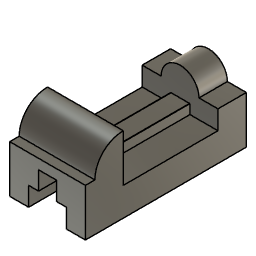
Robocon_Task1C_2 v1 (Autodesk Fusion 360 design; units mm, degrees)
Autodesk Fusion 360 part; units mm, degrees
sketch "Sketch1" plane through (0, 0, 0) normal (0, 0, 1) x (1, 0, 0) in component "Component"
  line L0 (40, -85) -> (-40, -85)
  line L1 (-40, -85) -> (-40, 85)
  line L2 (-40, 85) -> (40, 85)
  line L3 (40, 85) -> (40, -85)
  line L4 (40, -85) -> (-40, 85) construction
  line L5 (-40, -85) -> (40, 85) construction
  dimension "d1" = 80
  dimension "d2" = 170
  constraint horizontal L0
  constraint perpendicular L0 L1
  constraint parallel L0 L2
  constraint parallel L1 L3
  constraint coincident L4 origin
  constraint coincident L5 origin
  measures "d1" distance of L1.end L2.end
  measures "d2" distance of L0.end L1.end
extrude "Extrude1" add sketch "Sketch1" along normal blind 30 in component "Component"
sketch "Sketch2" plane through (0, 0, 30) normal (0, 0, 1) x (-1, 0, 0) in component "Component"
  line L0 (-40, -85) -> (40, -85)
  line L1 (40, -85) -> (40, 85)
  line L2 (40, 85) -> (-40, 85)
  line L3 (-40, 85) -> (-40, -85)
  line L4 (40, 75) -> (-40, 75)
  dimension "d5" = 10
  constraint coincident L1 L4.start
  constraint coincident L3 L4.end
  constraint perpendicular L3 L4
  measures "d5" distance of L2 L4
extrude "Extrude2" add sketch "Sketch2" along normal blind 20 contours L1 L2 L3 L4 in component "Component"
sketch "Sketch3" plane through (0, -85, 0) normal (0, -1, 0) x (1, 0, 0) in component "Component"
  line L0 (-40, 0) -> (40, 0)
  line L1 (40, 0) -> (40, 50)
  line L2 (40, 50) -> (-40, 50)
  line L3 (-40, 50) -> (-40, 0)
  line L4 (-20, 0) -> (-20, 20)
  line L5 (-20, 20) -> (-10, 20)
  line L6 (-10, 20) -> (-10, 40)
  line L7 (-10, 40) -> (10, 40)
  line L8 (10, 40) -> (10, 20)
  line L9 (10, 20) -> (20, 20)
  line L10 (20, 20) -> (20, 0)
  constraint coincident L0 L4.start
  constraint perpendicular L0 L4
  constraint perpendicular L4 L5
  constraint perpendicular L5 L6
  constraint perpendicular L6 L7
  constraint perpendicular L7 L8
  constraint perpendicular L8 L9
  constraint coincident L0 L10.end
  constraint perpendicular L0 L10
sketch "Sketch4" plane through (0, 0, 30) normal (0, 0, 1) x (-1, 0, 0) in component "Component"
  line L0 (40, 75) -> (-40, 75)
  line L1 (-40, 75) -> (-40, -85)
  line L2 (-40, -85) -> (40, -85)
  line L3 (40, -85) -> (40, 75)
  line L4 (40, -55) -> (-40, -55)
  dimension "d10" = 30
  constraint coincident L3 L4.start
  constraint perpendicular L3 L4
  measures "d10" distance of L2 L4
extrude "Extrude4" add sketch "Sketch4" along normal blind 40 contours L1 L2 L3 L4 in component "Component"
sketch "Sketch5" plane through (0, 55, 0) normal (0, -1, 0) x (1, 0, 0) in component "Component"
  line L0 (-40, 30) -> (40, 30)
  line L1 (40, 30) -> (40, 70)
  line L2 (40, 70) -> (-40, 70)
  line L3 (-40, 70) -> (-40, 30)
  circle A0 centre (0, 50) radius 20
  line L4 (-40, 50) -> (40, 50)
  dimension "d13" = 40
  dimension "d14" = 20
  constraint tangent L2 A0
  constraint midpoint L3 L4.start
  constraint midpoint L1 L4.end
  measures "d13" distance of L1 A0.centre
  measures "d14" distance of L2 A0.centre
extrude "Extrude5" cut sketch "Sketch5" against normal up to surface (30 mm away) contours L2 L3 A0 L4 | L1 L2 A0 L4 in component "Component"
sketch "Sketch6" plane through (0, 0, 30) normal (0, 0, 1) x (-1, 0, 0) in component "Component"
  line L0 (-40, -55) -> (40, -55)
  line L1 (40, -55) -> (40, 75)
  line L2 (40, 75) -> (-40, 75)
  line L3 (-40, 75) -> (-40, -55)
  line L4 (-40, 45) -> (40, 45)
  dimension "d17" = 30
  constraint coincident L3 L4.start
  constraint coincident L1 L4.end
  constraint perpendicular L1 L4
  measures "d17" distance of L2 L4
extrude "Extrude6" add sketch "Sketch6" along normal blind 50 contours L1 L2 L3 L4 in component "Component"
sketch "Sketch7" plane through (40, 0, 0) normal (1, 0, 0) x (0, 1, 0) in component "Component"
  line L0 (85, 50) -> (55, 50)
  line L1 (55, 50) -> (55, 30)
  line L2 (55, 30) -> (-45, 30)
  line L3 (-45, 30) -> (-45, 80)
  line L4 (-45, 80) -> (-75, 80)
  line L5 (-75, 80) -> (-75, 50)
  line L6 (-75, 50) -> (-85, 50)
  line L7 (-85, 50) -> (-85, 0)
  line L8 (-85, 0) -> (85, 0)
  line L9 (85, 0) -> (85, 50)
  circle A0 centre (-45, 50) radius 30
  dimension "d20" = 60
  constraint coincident L3 A0.centre
  constraint coincident L5.end A0
  measures "d20" diameter of A0
extrude "Extrude7" cut sketch "Sketch7" against normal up to surface (80 mm away) contours L4 L5 A0 in component "Component"
sketch "Sketch8" plane through (0, -85, 0) normal (0, -1, 0) x (1, 0, 0) in component "Component"
  line L0 (-40, 0) -> (40, 0)
  line L1 (40, 0) -> (40, 50)
  line L2 (40, 50) -> (-40, 50)
  line L3 (-40, 50) -> (-40, 0)
  line L4 (-20, 0) -> (-20, 20)
  line L5 (-20, 20) -> (-10, 20)
  line L6 (10, 20) -> (20, 20)
  line L7 (20, 20) -> (20, 0)
  line L8 (10, 20) -> (-10, 20)
  constraint coincident L0 L4.start
  constraint perpendicular L0 L4
  constraint perpendicular L4 L5
  constraint coincident L0 L7.end
  constraint perpendicular L0 L7
  constraint parallel L5 L8
extrude "Extrude8" cut sketch "Sketch8" against normal up to surface (170 mm away) contours L0 L4 L5 L6 L7 L8 in component "Component"
sketch "Sketch10" plane through (0, 0, 30) normal (0, 0, 1) x (-1, 0, 0) in component "Component"
  line L0 (40, 45) -> (-40, 45)
  line L1 (-40, 45) -> (-40, -55)
  line L2 (-40, -55) -> (40, -55)
  line L3 (40, -55) -> (40, 45)
  line L4 (-10.4269, -55) -> (-10.4269, 45)
  line L5 (9.8376, 45) -> (9.8376, -55)
  constraint coincident L2 L4.start
  constraint coincident L0 L4.end
  constraint perpendicular L0 L4
  constraint coincident L0 L5.start
  constraint coincident L2 L5.end
  constraint perpendicular L2 L5
extrude "Extrude9" add sketch "Sketch10" along normal blind 10 contours L0 L2 L4 L5 in component "Component"
sketch "Sketch13" plane through (0, -85, 0) normal (0, -1, 0) x (1, 0, 0) in component "Component"
  line L0 (-20, 0) -> (-20, 20)
  line L1 (-20, 20) -> (20, 20)
  line L2 (20, 20) -> (20, 0)
  line L3 (20, 0) -> (40, 0)
  line L4 (40, 0) -> (40, 50)
  line L5 (40, 50) -> (-40, 50)
  line L6 (-40, 50) -> (-40, 0)
  line L7 (-40, 0) -> (-20, 0)
  line L8 (-10, 20) -> (-10, 40)
  line L9 (-10, 40) -> (10, 40)
  line L10 (10, 40) -> (10, 20)
  line L11 (-9.5, 20) -> (-9.5, 39.5)
  line L12 (-9.5, 39.5) -> (9.5, 39.5)
  line L13 (9.5, 39.5) -> (9.5, 20)
  dimension "d38" = 0.5
  dimension "d39" = 0.5
  dimension "d40" = 0.5
  constraint coincident L1 L8.start
  constraint perpendicular L1 L8
  constraint perpendicular L8 L9
  constraint coincident L1 L10.end
  constraint perpendicular L1 L10
  constraint coincident L1 L11.start
  constraint perpendicular L1 L11
  constraint perpendicular L11 L12
  constraint coincident L1 L13.end
  constraint perpendicular L1 L13
  measures "d38" distance of L10 L13
  measures "d39" distance of L8 L11
  measures "d40" distance of L9 L12
extrude "Extrude10" cut sketch "Sketch13" against normal up to surface (170 mm away) contours L1 L11 L12 L13 in component "Component"
component "Component" placed x (1, 0, 0) y (0, 1, 0) z (0, 0, 1) at (0, 0, 0)
